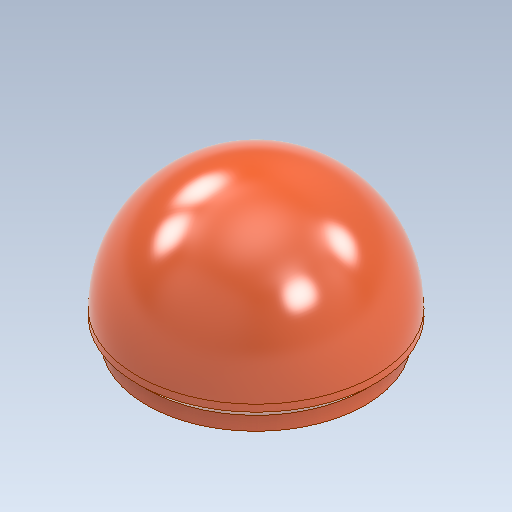
# Autodesk Inventor part: forward_endcap
Saved by Autodesk Inventor 2020.2 (Build 242310000, 310)
## iProperties
Created: 2019-11-09
Part Number: forward_endcap
Material: Wood (Birch)
Document SubType Name: Modeling
Designer: agmle
Density: 0.55 g/cm^3
Appearance: Smooth - Light Orange
Mass: 633.65 g
Surface Area: 1715.99 cm^2
Volume: 1152.09 cm^3
Author: agmle
Autodesk Inventor part; units mm, degrees
ref_plane "YZ Plane" through (0, 0, 0) normal (1, 0, 0) x (0, 1, 0)
ref_plane "XZ Plane" through (0, 0, 0) normal (0, 1, 0) x (-1, 0, 0)
ref_plane "XY Plane" through (0, 0, 0) normal (0, 0, 1) x (1, 0, 0)
sketch "Sketch1" plane through (0, 0, 0) normal (0, 0, 1) x (1, 0, 0)
  line L0 (0, 0) -> (0, 277.1469) construction
  line L1 (94.5134, 0) -> (100.8634, 0)
  line L2 (100.8634, 0) -> (100.8634, 12.7)
  line L3 (100.8634, 12.7) -> (109.5375, 12.7)
  line L4 (94.5134, 0) -> (94.5134, 27.7241)
  line L5 (109.5375, 12.7) -> (109.5375, -9.377) construction
  line L6 (109.5375, 12.7) -> (109.5375, 27.7241)
  line L7 (109.5375, 27.7241) -> (94.5134, 27.7241) construction
  arc A0 (94.5134, 27.7241) -> (0, 122.2375) centre (0, 27.7241) ccw
  arc A1 (109.5375, 27.7241) -> (0, 137.2616) centre (0, 27.7241) ccw
  line L8 (0, 137.2616) -> (0, 122.2375)
  dimension "d0" = 6.35
  dimension "d1" = 12.7
  dimension "d2" = 8.6741
  dimension "d3" = 100.8634
  dimension "d11" = 15.0241
  constraints: 18 end point, 5 vertical, 4 point on circle, 4 point on line, 3 perpendicular, 2 centre point, 1 coincident, 1 horizontal, 1 tangent
  measures "d0" distance of L1.start L1.end
  measures "d1" distance of L1.end L2.end
  measures "d2" distance of L2.end L3.end
  measures "d3" distance between parallel lines of L0 L2
  measures "d11" distance of L6.end L3.end
revolve "Revolution1" add sketch "Sketch1" angle 360 about axis through (0, 0, 0) along (0, 1, 0)
fillet "Fillet1" radius 3.175 1 edges at (-94.5134, 0, 0)
chamfer "Chamfer1" distance 8.6741 angle 45 1 edges at (-109.5375, 12.7, 0)
equation "\"d2\" = hull_wall"
equation "\"d3\" = 0.5 * hull_id"
equation "\"d8\" = hull_wall"
equation "\"hull_od\" = 219.075"
equation "\"hull_id\" = 201.7268"
equation "\"hull_wall\" = 8.6741"
equation "\"hull_length\" = 609.6"
equation "\"hull_spacing\" = 390.525"
equation "\"impeller_od\" = 76.2"
equation "\"impeller_clearance\" = 0.5"
equation "\"impeller_shaft_id\" = 3.175"
equation "\"impeller_shaft_od\" = 5.715"
equation "\"impeller_shaft_support\" = 3.175"
equation "\"impeller_intake_od\" = 19.05"
equation "\"impeller_vane_thick\" = 2"
equation "\"impeller_vane_inner_rad\" = 3.175"
equation "\"impeller_vane_outer_rad\" = 0.37206"
equation "\"magnet_od\" = 5.95"
equation "\"magnet_clearance\" = 0.25"
equation "\"magnet_rad\" = 0.25"
equation "\"magnet_circle_offset\" = 3.175"
equation "\"motor_shaft_od\" = 12.7"
equation "\"motor_shaft_length\" = 31.75"
equation "\"motor_shaft_key\" = 3.048"
equation "\"slab_thick\" = 34.671"
body "Solid1"
